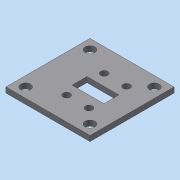
# Autodesk Inventor part: Part4
Saved by Autodesk Inventor 2016 SP1 (Build 200210100, 210)
## iProperties
Created: 2016-03-20
Part Number: Part4
Material: Generic
Document SubType Name: Modeling
Designer: Mohamed A.
Density: 1 g/cm^3
Appearance: Default
Author: Mohamed A.
Autodesk Inventor part; units mm, degrees
ref_plane "YZ Plane" through (0, 0, 0) normal (1, 0, 0) x (0, 1, 0)
ref_plane "XZ Plane" through (0, 0, 0) normal (0, 1, 0) x (-1, 0, 0)
ref_plane "XY Plane" through (0, 0, 0) normal (0, 0, 1) x (1, 0, 0)
sketch "Sketch1" plane through (0, 0, 0) normal (0, 0, 1) x (1, 0, 0)
  circle A0 centre (9.5006, -10.0358) radius 2
  circle A1 centre (-2.9994, -10.0358) radius 2
  circle A2 centre (-2.9994, 10.9642) radius 2
  circle A3 centre (9.5006, 10.9642) radius 2
  line L0 (9.0506, -3.7358) -> (6.9506, -3.7358)
  line L1 (6.9506, -3.7358) -> (-6.3494, -3.7358)
  line L2 (-6.3494, -3.7358) -> (-6.3494, 4.6642)
  line L3 (-6.3494, 4.6642) -> (11.5506, 4.6642)
  line L4 (11.5506, 4.6642) -> (11.5506, -3.7358)
  line L5 (11.5506, -3.7358) -> (9.0506, -3.7358)
  line L6 (9.0506, -3.7358) -> (9.0506, -8.5358) construction
  line L7 (9.0506, -8.5358) -> (6.9506, -8.5358) construction
  line L8 (6.9506, -8.5358) -> (6.9506, -3.7358) construction
  line L9 (-23.9494, 23.9642) -> (-23.9494, -23.0358)
  circle A4 centre (-18.4494, -17.5358) radius 1.4 construction
  circle A5 centre (-18.4494, 18.4642) radius 1.4 construction
  circle A6 centre (17.5506, 18.4642) radius 1.4 construction
  circle A7 centre (17.5506, -17.5358) radius 1.4 construction
  circle A8 centre (-18.4494, -17.5358) radius 1.4 construction
  circle A9 centre (17.5506, -17.5358) radius 1.4 construction
  circle A10 centre (17.5506, 18.4642) radius 1.4 construction
  circle A11 centre (-18.4494, 18.4642) radius 1.4 construction
  circle A12 centre (-2.9994, 10.9642) radius 0.9
  circle A13 centre (9.5006, 10.9642) radius 0.9
  circle A14 centre (9.5006, -10.0358) radius 0.9
  circle A15 centre (-2.9994, -10.0358) radius 0.9
  line L10 (-23.9494, -23.0358) -> (23.0506, -23.0358)
  line L11 (23.0506, -23.0358) -> (23.0506, 23.9642)
  line L12 (23.0506, 23.9642) -> (-23.9494, 23.9642)
  line L13 (10.4426, -23.0358) -> (10.4426, 23.9642) construction
  line L14 (-22.2241, 23.9642) -> (-22.2241, -23.0358) construction
  circle A16 centre (17.5506, -17.5358) radius 2.75
  circle A17 centre (-18.4494, -17.5358) radius 2.75
  circle A18 centre (17.5506, 18.4642) radius 2.75
  circle A19 centre (-18.4494, 18.4642) radius 2.75
  point P0 (0, 0)
extrude "Extrusion1" add sketch "Sketch1" along normal blind 3 contours L12 L11 L10 L9
body "Solid1"
